Autodesk Fusion 360 part; units mm, degrees
note: some values were not read from the file. Set by a fixed rule: which face or edge a step refers to.
(part 2 of 4)
sketch "Sketch5" plane through (0, 0, -9.6) normal (0, 0, -1) x (1, 0, 0) in component "M5xxx-base"
  line L0 (101.4, -66.4) -> (-101.4, -66.4) construction
  line L1 (-101.4, -66.4) -> (-101.4, 66.4) construction
  line L2 (-101.4, 66.4) -> (101.4, 66.4) construction
  line L3 (101.4, 66.4) -> (101.4, -66.4) construction
  line L4 (101.4, -66.4) -> (-101.4, 66.4) construction
  line L5 (-101.4, -66.4) -> (101.4, 66.4) construction
  line L6 (113.4, -70) -> (113.4, 70) construction
  line L7 (-107, -78.4) -> (106, -78.4) construction
  circle A0 centre (101.4, -66.4) radius 6
  circle A1 centre (101.4, 66.4) radius 6
  circle A2 centre (0, 66.4) radius 6
  circle A3 centre (0, -66.4) radius 6
  circle A4 centre (-101.4, -66.4) radius 6
  circle A5 centre (-101.4, 66.4) radius 6
  line L8 (-82, 62) -> (-10, 62)
  line L9 (-10, 62) -> (-10, 15)
  line L10 (-15, 10) -> (-82, 10)
  line L11 (-87, 15) -> (-87, 57)
  line L12 (10, 15) -> (10, 57)
  line L13 (15, 62) -> (82, 62)
  line L14 (87, 57) -> (87, 15)
  line L15 (82, 10) -> (15, 10)
  line L16 (-87, -57) -> (-87, -15)
  line L17 (-82, -10) -> (-15, -10)
  line L18 (-10, -15) -> (-10, -57)
  line L19 (-15, -62) -> (-82, -62)
  line L20 (87, -62) -> (15, -62)
  line L21 (10, -57) -> (10, -15)
  line L22 (15, -10) -> (87, -10)
  line L23 (87, -10) -> (87, -62)
  arc A6 (-15, 10) -> (-10, 15) centre (-15, 15) ccw
  arc A7 (-87, 15) -> (-82, 10) centre (-82, 15) ccw
  arc A8 (-82, 62) -> (-87, 57) centre (-82, 57) ccw
  arc A9 (15, 62) -> (10, 57) centre (15, 57) ccw
  arc A10 (87, 57) -> (82, 62) centre (82, 57) ccw
  arc A11 (82, 10) -> (87, 15) centre (82, 15) ccw
  arc A12 (10, 15) -> (15, 10) centre (15, 15) ccw
  arc A13 (-82, -10) -> (-87, -15) centre (-82, -15) ccw
  arc A14 (-10, -15) -> (-15, -10) centre (-15, -15) ccw
  arc A15 (-15, -62) -> (-10, -57) centre (-15, -57) ccw
  arc A16 (-87, -57) -> (-82, -62) centre (-82, -57) ccw
  arc A17 (10, -57) -> (15, -62) centre (15, -57) ccw
  arc A18 (15, -10) -> (10, -15) centre (15, -15) ccw
  line L24 (-107, -76.4) -> (106, -76.4)
  line L25 (106, 76.4) -> (-107, 76.4)
  arc A19 (-107, 76.4) -> (-113.3999, 69.9694) centre (-107, 70) ccw
  line L26 (-113.3999, 69.9694) -> (-113.3999, -69.9694)
  arc A20 (-113.3999, -69.9694) -> (-107, -76.4) centre (-107, -70) ccw
  arc A21 (106, -76.4) -> (112.4, -70) centre (106, -70) ccw
  line L27 (112.4, -70) -> (112.4, 70)
  arc A22 (112.4, 70) -> (106, 76.4) centre (106, 70) ccw
  arc A23 (-113.3999, -69.9694) -> (-107, -76.4) centre (-107, -70) ccw
  line L28 (-107, -76.4) -> (106, -76.4)
  arc A24 (106, -76.4) -> (112.4, -70) centre (106, -70) ccw
  line L29 (112.4, -70) -> (112.4, 70)
  arc A25 (112.4, 70) -> (106, 76.4) centre (106, 70) ccw
  line L30 (106, 76.4) -> (-107, 76.4)
  arc A26 (-107, 76.4) -> (-113.3999, 69.9694) centre (-107, 70) ccw
  line L31 (-113.3999, 69.9694) -> (-113.3999, -69.9694)
  line L32 (80.7624, -50) -> (85.3812, -42)
  line L33 (85.3812, -42) -> (94.6188, -42)
  line L34 (94.6188, -42) -> (99.2376, -50)
  line L35 (99.2376, -50) -> (94.6188, -58)
  line L36 (94.6188, -58) -> (85.3812, -58)
  line L37 (85.3812, -58) -> (80.7624, -50)
  line L38 (80.7624, 50) -> (85.3812, 58)
  line L39 (85.3812, 58) -> (94.6188, 58)
  line L40 (94.6188, 58) -> (99.2376, 50)
  line L41 (99.2376, 50) -> (94.6188, 42)
  line L42 (94.6188, 42) -> (85.3812, 42)
  line L43 (85.3812, 42) -> (80.7624, 50)
  line L44 (50.7624, -25) -> (55.3812, -17)
  line L45 (55.3812, -17) -> (64.6188, -17)
  line L46 (64.6188, -17) -> (69.2376, -25)
  line L47 (69.2376, -25) -> (64.6188, -33)
  line L48 (64.6188, -33) -> (55.3812, -33)
  line L49 (55.3812, -33) -> (50.7624, -25)
  line L50 (20.7624, 0) -> (25.3812, 8)
  line L51 (25.3812, 8) -> (34.6188, 8)
  line L52 (34.6188, 8) -> (39.2376, 0)
  line L53 (39.2376, 0) -> (34.6188, -8)
  line L54 (34.6188, -8) -> (25.3812, -8)
  line L55 (25.3812, -8) -> (20.7624, 0)
  line L56 (-9.2376, 25) -> (-4.6188, 33)
  line L57 (-4.6188, 33) -> (4.6188, 33)
  line L58 (4.6188, 33) -> (9.2376, 25)
  line L59 (9.2376, 25) -> (4.6188, 17)
  line L60 (4.6188, 17) -> (-4.6188, 17)
  line L61 (-4.6188, 17) -> (-9.2376, 25)
  line L62 (-39.2376, -50) -> (-34.6188, -42)
  line L63 (-34.6188, -42) -> (-25.3812, -42)
  line L64 (-25.3812, -42) -> (-20.7624, -50)
  line L65 (-20.7624, -50) -> (-25.3812, -58)
  line L66 (-25.3812, -58) -> (-34.6188, -58)
  line L67 (-34.6188, -58) -> (-39.2376, -50)
  line L68 (-39.2376, 50) -> (-34.6188, 58)
  line L69 (-34.6188, 58) -> (-25.3812, 58)
  line L70 (-25.3812, 58) -> (-20.7624, 50)
  line L71 (-20.7624, 50) -> (-25.3812, 42)
  line L72 (-25.3812, 42) -> (-34.6188, 42)
  line L73 (-34.6188, 42) -> (-39.2376, 50)
  line L74 (-69.2376, -25) -> (-64.6188, -17)
  line L75 (-64.6188, -17) -> (-55.3812, -17)
  line L76 (-55.3812, -17) -> (-50.7624, -25)
  line L77 (-50.7624, -25) -> (-55.3812, -33)
  line L78 (-55.3812, -33) -> (-64.6188, -33)
  line L79 (-64.6188, -33) -> (-69.2376, -25)
  line L80 (-99.2376, 0) -> (-94.6188, 8)
  line L81 (-94.6188, 8) -> (-85.3812, 8)
  line L82 (-85.3812, 8) -> (-80.7624, 0)
  line L83 (-80.7624, 0) -> (-85.3812, -8)
  line L84 (-85.3812, -8) -> (-94.6188, -8)
  line L85 (-94.6188, -8) -> (-99.2376, 0)
  line L86 (-99.2376, 25) -> (-94.6188, 33)
  line L87 (-94.6188, 33) -> (-85.3812, 33)
  line L88 (-85.3812, 33) -> (-80.7624, 25)
  line L89 (-80.7624, 25) -> (-85.3812, 17)
  line L90 (-85.3812, 17) -> (-94.6188, 17)
  line L91 (-94.6188, 17) -> (-99.2376, 25)
  line L92 (-69.2376, -50) -> (-64.6188, -42)
  line L93 (-64.6188, -42) -> (-55.3812, -42)
  line L94 (-55.3812, -42) -> (-50.7624, -50)
  line L95 (-50.7624, -50) -> (-55.3812, -58)
  line L96 (-55.3812, -58) -> (-64.6188, -58)
  line L97 (-64.6188, -58) -> (-69.2376, -50)
  line L98 (-69.2376, 50) -> (-64.6188, 58)
  line L99 (-64.6188, 58) -> (-55.3812, 58)
  line L100 (-55.3812, 58) -> (-50.7624, 50)
  line L101 (-50.7624, 50) -> (-55.3812, 42)
  line L102 (-55.3812, 42) -> (-64.6188, 42)
  line L103 (-64.6188, 42) -> (-69.2376, 50)
  line L104 (-39.2376, -25) -> (-34.6188, -17)
  line L105 (-34.6188, -17) -> (-25.3812, -17)
  line L106 (-25.3812, -17) -> (-20.7624, -25)
  line L107 (-20.7624, -25) -> (-25.3812, -33)
  line L108 (-25.3812, -33) -> (-34.6188, -33)
  line L109 (-34.6188, -33) -> (-39.2376, -25)
  line L110 (4.6188, 8) -> (9.2376, 0)
  line L111 (9.2376, 0) -> (4.6188, -8)
  line L112 (4.6188, -8) -> (-4.6188, -8)
  line L113 (-4.6188, -8) -> (-9.2376, 0)
  line L114 (-9.2376, 0) -> (-4.6188, 8)
  line L115 (-4.6188, 8) -> (4.6188, 8)
  line L116 (20.7624, 25) -> (25.3812, 33)
  line L117 (25.3812, 33) -> (34.6188, 33)
  line L118 (34.6188, 33) -> (39.2376, 25)
  line L119 (39.2376, 25) -> (34.6188, 17)
  line L120 (34.6188, 17) -> (25.3812, 17)
  line L121 (25.3812, 17) -> (20.7624, 25)
  line L122 (50.7624, -50) -> (55.3812, -42)
  line L123 (55.3812, -42) -> (64.6188, -42)
  line L124 (64.6188, -42) -> (69.2376, -50)
  line L125 (69.2376, -50) -> (64.6188, -58)
  line L126 (64.6188, -58) -> (55.3812, -58)
  line L127 (55.3812, -58) -> (50.7624, -50)
  line L128 (50.7624, 50) -> (55.3812, 58)
  line L129 (55.3812, 58) -> (64.6188, 58)
  line L130 (64.6188, 58) -> (69.2376, 50)
  line L131 (69.2376, 50) -> (64.6188, 42)
  line L132 (64.6188, 42) -> (55.3812, 42)
  line L133 (55.3812, 42) -> (50.7624, 50)
  line L134 (80.7624, -25) -> (85.3812, -17)
  line L135 (85.3812, -17) -> (94.6188, -17)
  line L136 (94.6188, -17) -> (99.2376, -25)
  line L137 (99.2376, -25) -> (94.6188, -33)
  line L138 (94.6188, -33) -> (85.3812, -33)
  line L139 (85.3812, -33) -> (80.7624, -25)
  line L140 (80.7624, 25) -> (85.3812, 33)
  line L141 (85.3812, 33) -> (94.6188, 33)
  line L142 (94.6188, 33) -> (99.2376, 25)
  line L143 (99.2376, 25) -> (94.6188, 17)
  line L144 (94.6188, 17) -> (85.3812, 17)
  line L145 (85.3812, 17) -> (80.7624, 25)
  line L146 (50.7624, 0) -> (55.3812, 8)
  line L147 (55.3812, 8) -> (64.6188, 8)
  line L148 (64.6188, 8) -> (69.2376, 0)
  line L149 (69.2376, 0) -> (64.6188, -8)
  line L150 (64.6188, -8) -> (55.3812, -8)
  line L151 (55.3812, -8) -> (50.7624, 0)
  line L152 (20.7624, -25) -> (25.3812, -17)
  line L153 (25.3812, -17) -> (34.6188, -17)
  line L154 (34.6188, -17) -> (39.2376, -25)
  line L155 (39.2376, -25) -> (34.6188, -33)
  line L156 (34.6188, -33) -> (25.3812, -33)
  line L157 (25.3812, -33) -> (20.7624, -25)
  line L158 (-9.2376, 50) -> (-4.6188, 58)
  line L159 (-4.6188, 58) -> (4.6188, 58)
  line L160 (4.6188, 58) -> (9.2376, 50)
  line L161 (9.2376, 50) -> (4.6188, 42)
  line L162 (4.6188, 42) -> (-4.6188, 42)
  line L163 (-4.6188, 42) -> (-9.2376, 50)
  line L164 (-9.2376, -50) -> (-4.6188, -42)
  line L165 (-4.6188, -42) -> (4.6188, -42)
  line L166 (4.6188, -42) -> (9.2376, -50)
  line L167 (9.2376, -50) -> (4.6188, -58)
  line L168 (4.6188, -58) -> (-4.6188, -58)
  line L169 (-4.6188, -58) -> (-9.2376, -50)
  line L170 (-39.2376, 25) -> (-34.6188, 33)
  line L171 (-34.6188, 33) -> (-25.3812, 33)
  line L172 (-25.3812, 33) -> (-20.7624, 25)
  line L173 (-20.7624, 25) -> (-25.3812, 17)
  line L174 (-25.3812, 17) -> (-34.6188, 17)
  line L175 (-34.6188, 17) -> (-39.2376, 25)
  line L176 (-69.2376, 0) -> (-64.6188, 8)
  line L177 (-64.6188, 8) -> (-55.3812, 8)
  line L178 (-55.3812, 8) -> (-50.7624, 0)
  line L179 (-50.7624, 0) -> (-55.3812, -8)
  line L180 (-55.3812, -8) -> (-64.6188, -8)
  line L181 (-64.6188, -8) -> (-69.2376, 0)
  line L182 (-99.2376, -25) -> (-94.6188, -17)
  line L183 (-94.6188, -17) -> (-85.3812, -17)
  line L184 (-85.3812, -17) -> (-80.7624, -25)
  line L185 (-80.7624, -25) -> (-85.3812, -33)
  line L186 (-85.3812, -33) -> (-94.6188, -33)
  line L187 (-94.6188, -33) -> (-99.2376, -25)
  line L188 (-99.2376, 50) -> (-94.6188, 58)
  line L189 (-94.6188, 58) -> (-85.3812, 58)
  line L190 (-85.3812, 58) -> (-80.7624, 50)
  line L191 (-80.7624, 50) -> (-85.3812, 42)
  line L192 (-85.3812, 42) -> (-94.6188, 42)
  line L193 (-94.6188, 42) -> (-99.2376, 50)
  line L194 (-99.2376, -50) -> (-94.6188, -42)
  line L195 (-94.6188, -42) -> (-85.3812, -42)
  line L196 (-85.3812, -42) -> (-80.7624, -50)
  line L197 (-80.7624, -50) -> (-85.3812, -58)
  line L198 (-85.3812, -58) -> (-94.6188, -58)
  line L199 (-94.6188, -58) -> (-99.2376, -50)
  line L200 (-69.2376, 25) -> (-64.6188, 33)
  line L201 (-64.6188, 33) -> (-55.3812, 33)
  line L202 (-55.3812, 33) -> (-50.7624, 25)
  line L203 (-50.7624, 25) -> (-55.3812, 17)
  line L204 (-55.3812, 17) -> (-64.6188, 17)
  line L205 (-64.6188, 17) -> (-69.2376, 25)
  line L206 (-39.2376, 0) -> (-34.6188, 8)
  line L207 (-34.6188, 8) -> (-25.3812, 8)
  line L208 (-25.3812, 8) -> (-20.7624, 0)
  line L209 (-20.7624, 0) -> (-25.3812, -8)
  line L210 (-25.3812, -8) -> (-34.6188, -8)
  line L211 (-34.6188, -8) -> (-39.2376, 0)
  line L212 (-9.2376, -25) -> (-4.6188, -17)
  line L213 (-4.6188, -17) -> (4.6188, -17)
  line L214 (4.6188, -17) -> (9.2376, -25)
  line L215 (9.2376, -25) -> (4.6188, -33)
  line L216 (4.6188, -33) -> (-4.6188, -33)
  line L217 (-4.6188, -33) -> (-9.2376, -25)
  line L218 (20.7624, 50) -> (25.3812, 58)
  line L219 (25.3812, 58) -> (34.6188, 58)
  line L220 (34.6188, 58) -> (39.2376, 50)
  line L221 (39.2376, 50) -> (34.6188, 42)
  line L222 (34.6188, 42) -> (25.3812, 42)
  line L223 (25.3812, 42) -> (20.7624, 50)
  line L224 (20.7624, -50) -> (25.3812, -42)
  line L225 (25.3812, -42) -> (34.6188, -42)
  line L226 (34.6188, -42) -> (39.2376, -50)
  line L227 (39.2376, -50) -> (34.6188, -58)
  line L228 (34.6188, -58) -> (25.3812, -58)
  line L229 (25.3812, -58) -> (20.7624, -50)
  line L230 (50.7624, 25) -> (55.3812, 33)
  line L231 (55.3812, 33) -> (64.6188, 33)
  line L232 (64.6188, 33) -> (69.2376, 25)
  line L233 (69.2376, 25) -> (64.6188, 17)
  line L234 (64.6188, 17) -> (55.3812, 17)
  line L235 (55.3812, 17) -> (50.7624, 25)
  line L236 (80.7624, 0) -> (85.3812, 8)
  line L237 (85.3812, 8) -> (94.6188, 8)
  line L238 (94.6188, 8) -> (99.2376, 0)
  line L239 (99.2376, 0) -> (94.6188, -8)
  line L240 (94.6188, -8) -> (85.3812, -8)
  line L241 (85.3812, -8) -> (80.7624, 0)
  dimension "d116" = 12
  dimension "d117" = 12
  dimension "d118" = 12
  constraint perpendicular L0 L1
  constraint parallel L0 L2
  constraint parallel L1 L3
  constraint horizontal L0
  constraint coincident L4 origin
  constraint coincident L5 origin
  constraint coincident L0.start L3.end
  constraint coincident L2.end L3.start
  constraint midpoint L2 A2.centre
  constraint midpoint L0 A3.centre
  constraint coincident L0.end L1.start
  constraint coincident L1.end L2.start
  constraint equal A3 A4
  constraint equal A0 A3
  constraint equal A0 A1
  constraint equal A1 A2
  constraint equal A2 A5
  measures "d116" distance of L3 L6
  measures "d117" distance of L0 L7
  measures "d118" diameter of A0
extrude "Extrude9" cut sketch "Sketch5" against normal blind 0.6 contours A0 | A1 | A2 | A3 | A4 | A5 bodies 3 in component "M5xxx-base"
combine "Combine1" operation cut target body 3 tool bodies 2 1 1 body 1 seen with x (1, 0, 0) y (0, 1, 0) z (0, 0, 1) at (0, 0, 16.6) body 1 seen with x (1, 0, 0) y (0, 1, 0) z (0, 0, 1) at (0, 0, 0) keep tools in component "M5xxx-base"
move_face "OffsetFaces1" offset -2 2 faces at (112.1333, -45.5056, 23.3243) (112.1333, -45.5056, 6.7243) on bodies 3 in component "M5xxx-base"
sketch "Sketch11" plane through (0, 0, 34.2) normal (0, 0, 1) x (-1, 0, 0) in component "M5xxx-base"
  line L0 (-88.8, 76) -> (-41.2, 76)
  line L1 (-41.2, 76) -> (-41.2, 78.4)
  line L2 (-41.2, 78.4) -> (-88.8, 78.4)
  line L3 (-88.8, 78.4) -> (-88.8, 76)
  line L4 (-65.4, 78.4) -> (-64.6, 78.4)
  line L5 (-64.6, 78.4) -> (-64.6, 76)
  line L6 (-64.6, 76) -> (-65.4, 76)
  line L7 (-65.4, 76) -> (-65.4, 78.4)
  line L8 (-65.4, 78.4) -> (-64.6, 76) construction
  line L9 (-64.6, 78.4) -> (-65.4, 76) construction
  line L10 (-65, 77.2) -> (-65, 76) construction
  point P0 (-65, 77.2)
  dimension "d193" = 0.8
  constraint perpendicular L4 L5
  constraint parallel L4 L6
  constraint parallel L5 L7
  constraint horizontal L4
  constraint coincident L2 L4.start
  constraint coincident L8 P0
  constraint coincident L9 P0
  constraint coincident L0 L6.end
  constraint coincident P0 L10.start
  constraint midpoint L0 L10.end
  constraint vertical L10
  measures "d193" distance of L5.end L6.end
extrude "Extrude17" add sketch "Sketch11" along normal blind 19 contours L0 L2 L4 L5 L6 L7 bodies 3 in component "M5xxx-base"
sketch "Sketch8" plane through (0, 0, -1.6) normal (0, 0, 1) x (-1, 0, 0) in component "M5xxx-base"
  line L0 (-111, 16.2) -> (-114.4, 16.2)
  line L1 (-114.4, 16.2) -> (-114.4, 15.4)
  line L2 (-114.4, 15.4) -> (-111, 15.4)
  line L3 (-111, 15.4) -> (-111, 16.2)
  line L4 (-111, 0.4) -> (-114.4, 0.4)
  line L5 (-114.4, 0.4) -> (-114.4, -0.4)
  line L6 (-114.4, -0.4) -> (-111, -0.4)
  line L7 (-111, -0.4) -> (-111, 0.4)
  line L8 (-111, -15.4) -> (-114.4, -15.4)
  line L9 (-114.4, -15.4) -> (-114.4, -16.2)
  line L10 (-114.4, -16.2) -> (-111, -16.2)
  line L11 (-111, -16.2) -> (-111, -15.4)
  line L12 (-111, 0) -> (-114.4, 0) construction
  circle A0 centre (-105, -70) radius 5
  line L13 (-106.5, -70) -> (-105.75, -68.701)
  line L14 (-105.75, -68.701) -> (-104.25, -68.701)
  line L15 (-104.25, -68.701) -> (-103.5, -70)
  line L16 (-103.5, -70) -> (-104.25, -71.299)
  line L17 (-104.25, -71.299) -> (-105.75, -71.299)
  line L18 (-105.75, -71.299) -> (-106.5, -70)
  circle A1 centre (-15, 70) radius 5
  line L19 (-15.75, 68.701) -> (-16.5, 70)
  line L20 (-16.5, 70) -> (-15.75, 71.299)
  line L21 (-15.75, 71.299) -> (-14.25, 71.299)
  line L22 (-14.25, 71.299) -> (-13.5, 70)
  line L23 (-13.5, 70) -> (-14.25, 68.701)
  line L24 (-14.25, 68.701) -> (-15.75, 68.701)
  circle A2 centre (105, -70) radius 5
  line L25 (104.25, -71.299) -> (103.5, -70)
  line L26 (103.5, -70) -> (104.25, -68.701)
  line L27 (104.25, -68.701) -> (105.75, -68.701)
  line L28 (105.75, -68.701) -> (106.5, -70)
  line L29 (106.5, -70) -> (105.75, -71.299)
  line L30 (105.75, -71.299) -> (104.25, -71.299)
  circle A3 centre (105, 70) radius 5
  line L31 (104.25, 68.701) -> (103.5, 70)
  line L32 (103.5, 70) -> (104.25, 71.299)
  line L33 (104.25, 71.299) -> (105.75, 71.299)
  line L34 (105.75, 71.299) -> (106.5, 70)
  line L35 (106.5, 70) -> (105.75, 68.701)
  line L36 (105.75, 68.701) -> (104.25, 68.701)
  circle A4 centre (-105, 70) radius 5
  line L37 (-105.75, 71.299) -> (-104.25, 71.299)
  line L38 (-104.25, 71.299) -> (-103.5, 70)
  line L39 (-103.5, 70) -> (-104.25, 68.701)
  line L40 (-104.25, 68.701) -> (-105.75, 68.701)
  line L41 (-105.75, 68.701) -> (-106.5, 70)
  line L42 (-106.5, 70) -> (-105.75, 71.299)
  dimension "d134" = 0.8
  dimension "d135" = 15
  constraint horizontal L0
  constraint vertical L1
  constraint horizontal L2
  constraint vertical L3
  constraint horizontal L4
  constraint vertical L5
  constraint horizontal L6
  constraint vertical L7
  constraint horizontal L8
  constraint vertical L9
  constraint horizontal L10
  constraint vertical L11
  constraint equal L7 L11
  constraint equal L3 L7
  constraint midpoint L7 L12.start
  constraint midpoint L5 L12.end
  constraint horizontal origin L12.start
  constraint symmetric L1.end L8.end L12
  measures "d134" distance of L0.start L2.end
  measures "d135" distance of L5.end L8.end
extrude "Extrude12" add sketch "Sketch8" along normal blind 44.8 contours L0 L1 L2 L3 | L4 L5 L6 L7 | L8 L9 L10 L11 bodies 3 in component "M5xxx-base"
chamfer "Chamfer7" distance 0.4 angle 45 41 edges at (114.4, -15.4, 37.4) (114.4, 0.4, 37.4) (114.4, 0.4, 37.4) (114.4, 0.4, 5.2) (114.4, 0.4, 21.8) (114.4, -15.4, 21.8) (114.4, -15.4, 5.2) (114.4, -15.4, 37.4) (114.4, 0.4, 37.4) (114.4, 0.4, 5.2) (114.4, 0.4, 21.8) (114.4, -15.4, 21.8) (114.4, -15.4, 5.2) (114.4, -15.4, 37.4) (114.4, 16.2, 37.4) (114.4, 16.2, 5.2) (114.4, 16.2, 21.8) (114.4, 16.2, 37.4) (114.4, 16.2, 5.2) (114.4, 16.2, 21.8) (114.4, 16.2, 37.4) (111, 15.4, 5.2) (111, 15.4, 37.4) (111, 15.4, 21.8) (111, 15.4, 5.2) (111, 15.4, 37.4) (111, 15.4, 21.8) (111, -0.4, 21.8) (111, -0.4, 37.4) (111, -0.4, 5.2) (111, -16.2, 5.2) (111, -16.2, 21.8) (111, -16.2, 37.4) (111, -16.2, 5.2) (111, -16.2, 21.8) (111, -16.2, 37.4) (111, -16.2, 37.4) (111, -0.4, 37.4) (111, 15.4, 37.4) (65.4, -78.4, 43.7) (64.6, -76, 43.7) measured on face at (114.4, 52, 12.8214) measured on face at (114.4, 52, 12.8214) measured on face at (114.4, 52, 12.8214) measured on face at (114.4, 52, 12.8214) measured on face at (114.4, 52, 12.8214) measured on face at (114.4, 52, 12.8214) measured on face at (114.4, 52, 12.8214) measured on face at (114.4, 52, 12.8214) measured on face at (114.4, 52, 12.8214) measured on face at (114.4, 52, 12.8214) measured on face at (114.4, 52, 12.8214) measured on face at (114.4, 52, 12.8214) measured on face at (114.4, 52, 12.8214) measured on face at (114.4, 52, 12.8214) measured on face at (114.4, 52, 12.8214) measured on face at (114.4, 52, 12.8214) measured on face at (114.4, 52, 12.8214) measured on face at (114.4, 52, 12.8214) measured on face at (114.4, 52, 12.8214) measured on face at (114.4, 52, 12.8214) measured on face at (114.4, 52, 12.8214) measured on face at (111, 52, 13.6667) measured on face at (111, 52, 13.6667) measured on face at (111, 52, 13.6667) measured on face at (111, 52, 13.6667) measured on face at (111, 52, 13.6667) measured on face at (111, 52, 13.6667) measured on face at (111, 52, 13.6667) measured on face at (111, 52, 13.6667) measured on face at (111, 52, 13.6667) measured on face at (111, 52, 13.6667) measured on face at (111, 52, 13.6667) measured on face at (111, 52, 13.6667) measured on face at (111, 52, 13.6667) measured on face at (111, 52, 13.6667) measured on face at (111, 52, 13.6667) measured on face at (111, 52, 13.6667) measured on face at (111, 52, 13.6667) measured on face at (111, 52, 13.6667) measured on face at (-64.8175, -78.4, 31.9138) measured on face at (-64.8175, -76, 32.7591) on bodies 3 in component "M5xxx-base"
sketch "Sketch7" plane through (114.4, 0, 0) normal (1, 0, 0) x (0, 1, 0) in component "M5xxx-base"
  line L0 (70, -6.1359) -> (70, 58.4)
  line L1 (70, 58.4) -> (-70, 58.4)
  line L2 (-70, 58.4) -> (-70, -6.1359)
  circle A0 centre (50, 7.5) radius 6.4
  line L3 (-61.6, 16.6) -> (-70, 16.6)
  line L4 (-75, 16.6) -> (-70, 16.6)
  line L5 (-75, 16.6) -> (-70, 16.6)
  line L6 (-70, 16.6) -> (-56, 16.6)
  line L7 (-56, 16.6) -> (-44, 16.6)
  line L8 (-44, 16.6) -> (-32, 16.6)
  line L9 (-58.4, 16.6) -> (-61.6, 16.6)
  line L10 (-71.75, 16.6) -> (-68.25, 16.6)
  line L11 (-71.75, 16.6) -> (-68.25, 16.6)
  line L12 (-71.75, 16.6) -> (-68.25, 16.6)
  line L13 (78.4, 58.4) -> (78.4, -6.1359)
  line L14 (50, 7.5) -> (56.4, 7.5) construction
  line L15 (47.7729, 13.5) -> (52.2271, 13.5)
  line L16 (47.7729, 1.5) -> (52.2271, 1.5)
  circle A1 centre (50, 7.5) radius 8
  line L17 (57.7859, 5.6614) -> (55, -6.1359)
  line L18 (42.2141, 5.6614) -> (45, -6.1359)
  line L19 (50, 7.5) -> (50, -6.1359) construction
  line L20 (46, 33.2) -> (54, 33.2)
  line L21 (50, 7.5) -> (50, 33.2) construction
  line L22 (15.8, 44) -> (32, 44)
  line L23 (32, 44) -> (32, 32.4)
  line L24 (32, 32.4) -> (15.8, 32.4)
  line L25 (15.8, 32.4) -> (15.8, 44)
  line L26 (15.8, 27) -> (32, 27)
  line L27 (32, 27) -> (32, 15.8)
  line L28 (32, 15.8) -> (15.8, 15.8)
  line L29 (15.8, 15.8) -> (15.8, 27)
  line L30 (15.8, 10.4) -> (32, 10.4)
  line L31 (32, 10.4) -> (32, -0.8)
  line L32 (32, -0.8) -> (15.8, -0.8)
  line L33 (15.8, -0.8) -> (15.8, 10.4)
  line L34 (-15.8, 10.4) -> (-0.4, 10.4)
  line L35 (-0.4, 10.4) -> (-0.4, -0.8)
  line L36 (-15.8, -0.8) -> (-15.8, 10.4)
  line L37 (0, 10.4) -> (15.4, 10.4)
  line L38 (15.4, 10.4) -> (15.4, -0.8)
  line L39 (0, -0.8) -> (0, 10.4)
  line L40 (-15.8, 27) -> (-0.4, 27)
  line L41 (-0.4, 27) -> (-0.4, 15.8)
  line L42 (-15.8, 15.8) -> (-15.8, 27)
  line L43 (0, 27) -> (15.4, 27)
  line L44 (15.4, 27) -> (15.4, 15.8)
  line L45 (0, 15.8) -> (0, 27)
  line L46 (0, 44) -> (15.4, 44)
  line L47 (15.4, 44) -> (15.4, 32.4)
  line L48 (0, 32.4) -> (0, 44)
  line L49 (-15.8, 44) -> (-0.4, 44)
  line L50 (-0.4, 44) -> (-0.4, 32.4)
  line L51 (-15.8, 32.4) -> (-15.8, 44)
  line L52 (-32, -0.8) -> (-32, 10.4)
  line L53 (-32, 10.4) -> (-16.2, 10.4)
  line L54 (-16.2, 10.4) -> (-16.2, -0.8)
  line L55 (-32, 15.8) -> (-32, 27)
  line L56 (-32, 27) -> (-16.2, 27)
  line L57 (-16.2, 27) -> (-16.2, 15.8)
  line L58 (-16.2, 44) -> (-16.2, 32.4)
  line L59 (-32, 32.4) -> (-32, 44)
  line L60 (-32, 44) -> (-16.2, 44)
  line L61 (-70, -6.1359) -> (70, -6.1359)
  line L62 (70, -6.1359) -> (70, 58.4)
  line L63 (70, 58.4) -> (-70, 58.4)
  line L64 (-70, 58.4) -> (-70, -6.1359)
  arc A2 (54, 34.2) -> (59, 39.2) centre (54, 39.2) ccw
  line L65 (54, 34.2) -> (46, 34.2)
  arc A3 (41, 39.2) -> (46, 34.2) centre (46, 39.2) ccw
  line L66 (41, 39.2) -> (41, 48.2)
  arc A4 (46, 53.2) -> (41, 48.2) centre (46, 48.2) ccw
  line L67 (46, 53.2) -> (54, 53.2)
  arc A5 (59, 48.2) -> (54, 53.2) centre (54, 48.2) ccw
  line L68 (59, 48.2) -> (59, 39.2)
  circle A6 centre (-50, 24.1) radius 6.5
  circle A7 centre (-50, 7.5) radius 6.5
  line L69 (45, -6.1359) -> (55, -6.1359)
  line L70 (-0.4, -0.8) -> (-15.8, -0.8)
  line L71 (15.4, -0.8) -> (0, -0.8)
  line L72 (-0.4, 15.8) -> (-15.8, 15.8)
  line L73 (15.4, 15.8) -> (0, 15.8)
  line L74 (-16.2, -0.8) -> (-32, -0.8)
  line L75 (-16.2, 15.8) -> (-32, 15.8)
  line L76 (15.4, 32.4) -> (0, 32.4)
  line L77 (-0.4, 32.4) -> (-15.8, 32.4)
  line L78 (-16.2, 32.4) -> (-32, 32.4)
  line L79 (15.4, 32.4) -> (15.8, 32.4)
  line L80 (15.8, 32.4) -> (15.8, 44)
  line L81 (15.4, 15.8) -> (15.8, 15.8)
  line L82 (15.8, 15.8) -> (15.8, 27)
  line L83 (15.4, -0.8) -> (15.8, -0.8)
  line L84 (15.8, -0.8) -> (15.8, 10.4)
  line L85 (0, 10.4) -> (-0.4, 10.4)
  line L86 (-0.4, 10.4) -> (-0.4, -0.8)
  line L87 (-16.2, -0.8) -> (-15.8, -0.8)
  line L88 (-15.8, -0.8) -> (-15.8, 10.4)
  line L89 (15.8, 10.4) -> (15.4, 10.4)
  line L90 (15.4, 10.4) -> (15.4, -0.8)
  line L91 (-0.4, -0.8) -> (0, -0.8)
  line L92 (0, -0.8) -> (0, 10.4)
  line L93 (0, 27) -> (-0.4, 27)
  line L94 (-0.4, 27) -> (-0.4, 15.8)
  line L95 (-16.2, 15.8) -> (-15.8, 15.8)
  line L96 (-15.8, 15.8) -> (-15.8, 27)
  line L97 (15.8, 27) -> (15.4, 27)
  line L98 (15.4, 27) -> (15.4, 15.8)
  line L99 (-0.4, 15.8) -> (0, 15.8)
  line L100 (0, 15.8) -> (0, 27)
  line L101 (15.8, 44) -> (15.4, 44)
  line L102 (15.4, 44) -> (15.4, 32.4)
  line L103 (-0.4, 32.4) -> (0, 32.4)
  line L104 (0, 32.4) -> (0, 44)
  line L105 (0, 44) -> (-0.4, 44)
  line L106 (-0.4, 44) -> (-0.4, 32.4)
  line L107 (-16.2, 32.4) -> (-15.8, 32.4)
  line L108 (-15.8, 32.4) -> (-15.8, 44)
  line L109 (-15.8, 10.4) -> (-16.2, 10.4)
  line L110 (-16.2, 10.4) -> (-16.2, -0.8)
  line L111 (-15.8, 27) -> (-16.2, 27)
  line L112 (-16.2, 27) -> (-16.2, 15.8)
  line L113 (-16.2, 44) -> (-16.2, 32.4)
  line L114 (-15.8, 44) -> (-16.2, 44)
  line L115 (75, 0) -> (-75, 0)
  circle A8 centre (-50, 6.5) radius 6.5
  line L116 (-32, 0) -> (-32, 10.4)
  line L117 (15.8, 10.4) -> (32, 10.4)
  line L118 (32, 10.4) -> (32, 0)
  circle A9 centre (-50, 23.1) radius 6.5
  line L119 (-32, 16.6) -> (-32, 27)
  line L120 (15.8, 27) -> (32, 27)
  line L121 (32, 27) -> (32, 16.6)
  arc A10 (54, 34.2) -> (59, 39.2) centre (54, 39.2) ccw
  line L122 (54, 34.2) -> (46, 34.2)
  arc A11 (41, 39.2) -> (46, 34.2) centre (46, 39.2) ccw
  line L123 (41, 39.2) -> (41, 48.2)
  arc A12 (46, 53.2) -> (41, 48.2) centre (46, 48.2) ccw
  line L124 (46, 53.2) -> (54, 53.2)
  arc A13 (59, 48.2) -> (54, 53.2) centre (54, 48.2) ccw
  line L125 (59, 48.2) -> (59, 39.2)
  line L126 (32, 43.6) -> (32, 31.6)
  line L127 (32, 31.6) -> (15.8, 31.6)
  line L128 (-32, 31.6) -> (-32, 43.6)
  line L129 (-32, 43.6) -> (32, 43.6)
  line L130 (-70, -6.1359) -> (70, -6.1359)
  line L131 (70, -6.1359) -> (70, 58.4)
  line L132 (70, 58.4) -> (-70, 58.4)
  line L133 (-70, 58.4) -> (-70, -6.1359)
  line L134 (15.8, 31.6) -> (15.8, 43.2)
  line L135 (15.8, 16.6) -> (15.8, 27)
  line L136 (15.8, 0) -> (15.8, 10.4)
  line L137 (-15.8, 10.4) -> (-0.4, 10.4)
  line L138 (-0.4, 10.4) -> (-0.4, 0)
  line L139 (-15.8, 31.6) -> (-15.8, 43.2)
  line L140 (0, 10.4) -> (15.4, 10.4)
  line L141 (15.4, 10.4) -> (15.4, 0)
  line L142 (0, 31.6) -> (0, 43.2)
  line L143 (-15.8, 27) -> (-0.4, 27)
  line L144 (-15.8, 16.6) -> (-15.8, 27)
  line L145 (0, 27) -> (15.4, 27)
  line L146 (0, 16.6) -> (0, 27)
  line L147 (15.4, 43.2) -> (15.4, 31.6)
  line L148 (15.4, 31.6) -> (0, 31.6)
  line L149 (-0.4, 43.2) -> (-0.4, 31.6)
  line L150 (-0.4, 31.6) -> (-15.8, 31.6)
  line L151 (-32, 10.4) -> (-16.2, 10.4)
  line L152 (-16.2, 10.4) -> (-16.2, 0)
  line L153 (-32, 27) -> (-16.2, 27)
  line L154 (-16.2, 43.2) -> (-16.2, 31.6)
  line L155 (-16.2, 31.6) -> (-32, 31.6)
  line L156 (15.8, 43.2) -> (15.4, 43.2)
  line L157 (0, 43.2) -> (-0.4, 43.2)
  line L158 (-15.8, 43.2) -> (-16.2, 43.2)
  line L159 (32, 16.6) -> (15.8, 16.6)
  line L160 (32, 0) -> (15.8, 0)
  line L161 (-0.4, 0) -> (-15.8, 0)
  line L162 (-15.8, 0) -> (-15.8, 10.4)
  line L163 (-0.4, 27) -> (-0.4, 16.6)
  line L164 (-0.4, 16.6) -> (-15.8, 16.6)
  line L165 (15.4, 0) -> (0, 0)
  line L166 (0, 0) -> (0, 10.4)
  line L167 (15.4, 27) -> (15.4, 16.6)
  line L168 (15.4, 16.6) -> (0, 16.6)
  line L169 (-16.2, 0) -> (-32, 0)
  line L170 (-16.2, 16.6) -> (-32, 16.6)
  line L171 (-16.2, 27) -> (-16.2, 16.6)
  dimension "d123" = 12
  dimension "d124" = 12.8
  dimension "d127" = 16
  dimension "d128" = 10
  dimension "d200" = 7.5
  constraint coincident A0.centre L14.start
  constraint coincident A0 L14.end
  constraint horizontal L14
  constraint coincident A0 L15.start
  constraint coincident A0 L15.end
  constraint horizontal L15
  constraint coincident A0 L16.start
  constraint coincident A0 L16.end
  constraint parallel L15 L16
  constraint symmetric L14 L15.end L16.end
  constraint concentric A0 A1
  constraint coincident A1 L17.start
  constraint coincident A1 L18.start
  constraint tangent A1 L18
  constraint tangent A1 L17
  constraint symmetric L17.end L18.end L19
  constraint midpoint L20 L21.end
  constraint perpendicular L20 L21
  constraint vertical L19
  constraint midpoint L19.end L69
  constraint coincident L17.end L61
  measures "d123" distance of L15 L16
  measures "d124" diameter of A0
  measures "d127" diameter of A1
  measures "d128" distance of L17.end L18.end
  measures "d200" distance of A0.centre L115
extrude "Extrude14" add sketch "Sketch7" along normal blind 2.4 contours A1 L17 L18 L61 L69 L115 L130 | A1 L17 L115 | A1 L115 | A1 L115 | A1 L18 L115 | A0 L15 | A0 L16 bodies 3 in component "M5xxx-base"
extrude "Extrude15" cut sketch "Sketch7" against normal blind 11 contours A0 L15 L16 bodies 3 in component "M5xxx-base"
sketch "Sketch12" plane through (111, 0, 0) normal (-1, 0, 0) x (0, -1, 0) in component "M5xxx-base"
  line L0 (-47.7729, 1.5) -> (-52.2271, 1.5)
  arc A0 (-52.2271, 13.5) -> (-52.2271, 1.5) centre (-50, 7.5) ccw
  line L1 (-52.2271, 13.5) -> (-47.7729, 13.5)
  arc A1 (-47.7729, 1.5) -> (-47.7729, 13.5) centre (-50, 7.5) ccw
  line L2 (-0.4, 43.2) -> (-0.4, 31.6)
  line L3 (-0.4, 31.6) -> (-15.8, 31.6)
  line L4 (-15.8, 31.6) -> (-15.8, 43.2)
  line L5 (15.4, 43.2) -> (15.4, 31.6)
  line L6 (15.4, 31.6) -> (0, 31.6)
  line L7 (0, 31.6) -> (0, 43.2)
  line L8 (32, 43.6) -> (32, 31.6)
  line L9 (32, 31.6) -> (15.8, 31.6)
  line L10 (15.8, 31.6) -> (15.8, 43.2)
  line L11 (15.8, 10.4) -> (32, 10.4)
  line L12 (32, 10.4) -> (32, 0)
  line L13 (15.8, 0) -> (15.8, 10.4)
  line L14 (15.8, 27) -> (32, 27)
  line L15 (32, 27) -> (32, 16.6)
  line L16 (15.8, 16.6) -> (15.8, 27)
  line L17 (0, 27) -> (15.4, 27)
  line L18 (0, 16.6) -> (0, 27)
  line L19 (-15.8, 27) -> (-0.4, 27)
  line L20 (-15.8, 16.6) -> (-15.8, 27)
  line L21 (-15.8, 10.4) -> (-0.4, 10.4)
  line L22 (-15.8, 0) -> (-15.8, 10.4)
  line L23 (-32, 0) -> (-32, 10.4)
  line L24 (-32, 10.4) -> (-16.2, 10.4)
  line L25 (-16.2, 27) -> (-16.2, 16.6)
  line L26 (-32, 16.6) -> (-32, 27)
  line L27 (-32, 27) -> (-16.2, 27)
  line L28 (-16.2, 43.2) -> (-16.2, 31.6)
  line L29 (-16.2, 31.6) -> (-32, 31.6)
  line L30 (-32, 31.6) -> (-32, 43.6)
  line L31 (-32, 43.6) -> (32, 43.6)
  circle A2 centre (50, 6.5) radius 6.5
  circle A3 centre (50, 23.1) radius 6.5
  arc A4 (-59, 39.2) -> (-54, 34.2) centre (-54, 39.2) ccw
  line L32 (-59, 39.2) -> (-59, 48.2)
  arc A5 (-54, 53.2) -> (-59, 48.2) centre (-54, 48.2) ccw
  line L33 (-54, 53.2) -> (-46, 53.2)
  arc A6 (-41, 48.2) -> (-46, 53.2) centre (-46, 48.2) ccw
  line L34 (-41, 48.2) -> (-41, 39.2)
  arc A7 (-46, 34.2) -> (-41, 39.2) centre (-46, 39.2) ccw
  line L35 (-46, 34.2) -> (-54, 34.2)
  line L36 (-70, -3.6) -> (70, -3.6)
  line L37 (70, -3.6) -> (70, 58.4)
  line L38 (70, 58.4) -> (-70, 58.4)
  line L39 (-70, 58.4) -> (-70, -3.6)
  circle A8 centre (-50, 7.5) radius 8.5
  line L40 (32, 0) -> (15.8, 0)
  line L41 (15.8, 43.2) -> (15.4, 43.2)
  line L42 (0, 43.2) -> (-0.4, 43.2)
  line L43 (-15.8, 43.2) -> (-16.2, 43.2)
  line L44 (32, 16.6) -> (15.8, 16.6)
  line L45 (0, 10.4) -> (15.4, 10.4)
  line L46 (15.4, 10.4) -> (15.4, 0)
  line L47 (15.4, 0) -> (0, 0)
  line L48 (0, 0) -> (0, 10.4)
  line L49 (15.4, 27) -> (15.4, 16.6)
  line L50 (15.4, 16.6) -> (0, 16.6)
  line L51 (-16.2, 16.6) -> (-32, 16.6)
  line L52 (-16.2, 0) -> (-32, 0)
  line L53 (-16.2, 10.4) -> (-16.2, 0)
  line L54 (-0.4, 10.4) -> (-0.4, 0)
  line L55 (-0.4, 0) -> (-15.8, 0)
  line L56 (-0.4, 27) -> (-0.4, 16.6)
  line L57 (-0.4, 16.6) -> (-15.8, 16.6)
  dimension "d201" = 17
  constraint concentric A0 A8
  measures "d201" diameter of A8
extrude "Extrude18" cut sketch "Sketch12" against normal blind 2.4 contours A8 bodies 3 in component "M5xxx-base"
chamfer "Chamfer14" distance 4 angle 30 1 edges at (116.8, 50, -6.1359) measured on face at (116.8, 50.7424, -3.5906) on bodies 3 in component "M5xxx-base"
sketch "Sketch14" plane through (-115.3999, 0, 0) normal (-1, 0, 0) x (0, -1, 0) in component "M5xxx-base"
  circle A0 centre (60, 7.5) radius 1.75
  circle A1 centre (60, 24.1) radius 1.75
  line L0 (-69.9653, -6.1359) -> (69.9653, -6.1359)
  line L1 (69.9653, -6.1359) -> (69.9653, 58.4)
  line L2 (69.9653, 58.4) -> (-69.9653, 58.4)
  line L3 (-69.9653, 58.4) -> (-69.9653, -6.1359)
  line L4 (0, 0) -> (0, 58.4) construction
  line L5 (6.9282, 22.6) -> (3.4641, 28.6)
  line L6 (3.4641, 28.6) -> (-3.4641, 28.6)
  line L7 (-3.4641, 28.6) -> (-6.9282, 22.6)
  line L8 (-6.9282, 22.6) -> (-3.4641, 16.6)
  line L9 (-3.4641, 16.6) -> (3.4641, 16.6)
  line L10 (3.4641, 16.6) -> (6.9282, 22.6)
  line L11 (-26.5359, 12) -> (-33.4641, 12)
  line L12 (-33.4641, 12) -> (-36.9282, 6)
  line L13 (-36.9282, 6) -> (-33.4641, 0)
  line L14 (-33.4641, 0) -> (-26.5359, 0)
  line L15 (-26.5359, 0) -> (-23.0718, 6)
  line L16 (-23.0718, 6) -> (-26.5359, 12)
  line L17 (3.4641, 12) -> (-3.4641, 12)
  line L18 (-3.4641, 12) -> (-6.9282, 6)
  line L19 (-6.9282, 6) -> (-3.4641, 0)
  line L20 (-3.4641, 0) -> (3.4641, 0)
  line L21 (3.4641, 0) -> (6.9282, 6)
  line L22 (6.9282, 6) -> (3.4641, 12)
  line L23 (33.4641, 12) -> (26.5359, 12)
  line L24 (26.5359, 12) -> (23.0718, 6)
  line L25 (23.0718, 6) -> (26.5359, 0)
  line L26 (26.5359, 0) -> (33.4641, 0)
  line L27 (33.4641, 0) -> (36.9282, 6)
  line L28 (36.9282, 6) -> (33.4641, 12)
  line L29 (-26.5359, 28.6) -> (-33.4641, 28.6)
  line L30 (-33.4641, 28.6) -> (-36.9282, 22.6)
  line L31 (-36.9282, 22.6) -> (-33.4641, 16.6)
  line L32 (-33.4641, 16.6) -> (-26.5359, 16.6)
  line L33 (-26.5359, 16.6) -> (-23.0718, 22.6)
  line L34 (-23.0718, 22.6) -> (-26.5359, 28.6)
  line L35 (33.4641, 28.6) -> (26.5359, 28.6)
  line L36 (26.5359, 28.6) -> (23.0718, 22.6)
  line L37 (23.0718, 22.6) -> (26.5359, 16.6)
  line L38 (26.5359, 16.6) -> (33.4641, 16.6)
  line L39 (33.4641, 16.6) -> (36.9282, 22.6)
  line L40 (36.9282, 22.6) -> (33.4641, 28.6)
  line L41 (-26.5359, 45.2) -> (-33.4641, 45.2)
  line L42 (-33.4641, 45.2) -> (-36.9282, 39.2)
  line L43 (-36.9282, 39.2) -> (-33.4641, 33.2)
  line L44 (-33.4641, 33.2) -> (-26.5359, 33.2)
  line L45 (-26.5359, 33.2) -> (-23.0718, 39.2)
  line L46 (-23.0718, 39.2) -> (-26.5359, 45.2)
  line L47 (3.4641, 45.2) -> (-3.4641, 45.2)
  line L48 (-3.4641, 45.2) -> (-6.9282, 39.2)
  line L49 (-6.9282, 39.2) -> (-3.4641, 33.2)
  line L50 (-3.4641, 33.2) -> (3.4641, 33.2)
  line L51 (3.4641, 33.2) -> (6.9282, 39.2)
  line L52 (6.9282, 39.2) -> (3.4641, 45.2)
  line L53 (33.4641, 45.2) -> (26.5359, 45.2)
  line L54 (26.5359, 45.2) -> (23.0718, 39.2)
  line L55 (23.0718, 39.2) -> (26.5359, 33.2)
  line L56 (26.5359, 33.2) -> (33.4641, 33.2)
  line L57 (33.4641, 33.2) -> (36.9282, 39.2)
  line L58 (36.9282, 39.2) -> (33.4641, 45.2)
  point P0 (0, 22.6)
  dimension "d221" = 6
  dimension "d224" = 30
  dimension "d225" = 16.6
  constraint coincident L4.start origin
  constraint midpoint L2 L4.end
  constraint horizontal L9
  constraint coincident L4 P0
  constraint coincident L4.start L20
  measures "d221" distance of P0 L10
extrude "Extrude21" cut sketch "Sketch14" against normal blind 2.4 contours L5 L6 L7 L8 L9 L10 | L11 L12 L13 L14 L15 L16 | L17 L18 L19 L20 L21 L22 | L23 L24 L25 L26 L27 L28 | L29 L30 L31 L32 L33 L34 | L35 L36 L37 L38 L39 L40 | L41 L42 L43 L44 L45 L46 | L47 L48 L49 L50 L51 L52 | L53 L54 L55 L56 L57 L58 bodies 3 in component "M5xxx-base"
sketch "Sketch15" plane through (0, -78.4, 0) normal (0, -1, 0) x (1, 0, 0) in component "M5xxx-base"
  line L0 (65, 53.2) -> (88.8, 53.2)
  arc A0 (93.8, 48.2) -> (88.8, 53.2) centre (88.8, 48.2) ccw
  line L1 (93.8, 48.2) -> (93.8, 39.2)
  arc A1 (88.8, 34.2) -> (93.8, 39.2) centre (88.8, 39.2) ccw
  line L2 (88.8, 34.2) -> (65, 34.2)
  line L3 (65, 34.2) -> (65, 53.2)
  line L4 (64.6, 34.2) -> (41.2, 34.2)
  arc A2 (36.2, 39.2) -> (41.2, 34.2) centre (41.2, 39.2) ccw
  line L5 (36.2, 39.2) -> (36.2, 48.2)
  arc A3 (41.2, 53.2) -> (36.2, 48.2) centre (41.2, 48.2) ccw
  line L6 (41.2, 53.2) -> (64.6, 53.2)
  line L7 (64.6, 53.2) -> (64.6, 34.2)
  arc A4 (32.6, 42) -> (32.6, 45.8) centre (32.6, 43.9) ccw
  line L8 (32.6, 42) -> (21.4, 42)
  arc A5 (21.4, 45.8) -> (21.4, 42) centre (21.4, 43.9) ccw
  line L9 (21.4, 45.8) -> (32.6, 45.8)
  line L10 (-107, -6.1359) -> (106, -6.1359)
  line L11 (106, -6.1359) -> (106, 58.4)
  line L12 (106, 58.4) -> (-107, 58.4)
  line L13 (-107, 58.4) -> (-107, -6.1359)
  line L14 (-86.6077, 6) -> (-90.0718, 12)
  line L15 (-90.0718, 12) -> (-97, 12)
  line L16 (-97, 12) -> (-100.4641, 6)
  line L17 (-100.4641, 6) -> (-97, 0)
  line L18 (-97, 0) -> (-90.0718, 0)
  line L19 (-90.0718, 0) -> (-86.6077, 6)
  line L20 (-70.4641, 6) -> (-67, 0)
  line L21 (-67, 12) -> (-70.4641, 6)
  line L22 (-60.0718, 12) -> (-67, 12)
  line L23 (-56.6077, 6) -> (-60.0718, 12)
  line L24 (-60.0718, 0) -> (-56.6077, 6)
  line L25 (-67, 0) -> (-60.0718, 0)
  line L26 (-40.4641, 6) -> (-37, 0)
  line L27 (-37, 12) -> (-40.4641, 6)
  line L28 (-30.0718, 12) -> (-37, 12)
  line L29 (-26.6077, 6) -> (-30.0718, 12)
  line L30 (-30.0718, 0) -> (-26.6077, 6)
  line L31 (-37, 0) -> (-30.0718, 0)
  line L32 (-10.4641, 6) -> (-7, 0)
  line L33 (-7, 12) -> (-10.4641, 6)
  line L34 (-0.0718, 12) -> (-7, 12)
  line L35 (3.3923, 6) -> (-0.0718, 12)
  line L36 (-0.0718, 0) -> (3.3923, 6)
  line L37 (-7, 0) -> (-0.0718, 0)
  line L38 (-100.4641, 22.6) -> (-97, 16.6)
  line L39 (-97, 28.6) -> (-100.4641, 22.6)
  line L40 (-90.0718, 28.6) -> (-97, 28.6)
  line L41 (-86.6077, 22.6) -> (-90.0718, 28.6)
  line L42 (-90.0718, 16.6) -> (-86.6077, 22.6)
  line L43 (-97, 16.6) -> (-90.0718, 16.6)
  line L44 (-70.4641, 22.6) -> (-67, 16.6)
  line L45 (-67, 28.6) -> (-70.4641, 22.6)
  line L46 (-60.0718, 28.6) -> (-67, 28.6)
  line L47 (-56.6077, 22.6) -> (-60.0718, 28.6)
  line L48 (-60.0718, 16.6) -> (-56.6077, 22.6)
  line L49 (-67, 16.6) -> (-60.0718, 16.6)
  line L50 (-40.4641, 22.6) -> (-37, 16.6)
  line L51 (-37, 28.6) -> (-40.4641, 22.6)
  line L52 (-30.0718, 28.6) -> (-37, 28.6)
  line L53 (-26.6077, 22.6) -> (-30.0718, 28.6)
  line L54 (-30.0718, 16.6) -> (-26.6077, 22.6)
  line L55 (-37, 16.6) -> (-30.0718, 16.6)
  line L56 (-10.4641, 22.6) -> (-7, 16.6)
  line L57 (-7, 28.6) -> (-10.4641, 22.6)
  line L58 (-0.0718, 28.6) -> (-7, 28.6)
  line L59 (3.3923, 22.6) -> (-0.0718, 28.6)
  line L60 (-0.0718, 16.6) -> (3.3923, 22.6)
  line L61 (-7, 16.6) -> (-0.0718, 16.6)
  line L62 (-100.4641, 39.2) -> (-97, 33.2)
  line L63 (-97, 45.2) -> (-100.4641, 39.2)
  line L64 (-90.0718, 45.2) -> (-97, 45.2)
  line L65 (-86.6077, 39.2) -> (-90.0718, 45.2)
  line L66 (-90.0718, 33.2) -> (-86.6077, 39.2)
  line L67 (-97, 33.2) -> (-90.0718, 33.2)
  line L68 (-70.4641, 39.2) -> (-67, 33.2)
  line L69 (-67, 45.2) -> (-70.4641, 39.2)
  line L70 (-60.0718, 45.2) -> (-67, 45.2)
  line L71 (-56.6077, 39.2) -> (-60.0718, 45.2)
  line L72 (-60.0718, 33.2) -> (-56.6077, 39.2)
  line L73 (-67, 33.2) -> (-60.0718, 33.2)
  line L74 (-40.4641, 39.2) -> (-37, 33.2)
  line L75 (-37, 45.2) -> (-40.4641, 39.2)
  line L76 (-30.0718, 45.2) -> (-37, 45.2)
  line L77 (-26.6077, 39.2) -> (-30.0718, 45.2)
  line L78 (-30.0718, 33.2) -> (-26.6077, 39.2)
  line L79 (-37, 33.2) -> (-30.0718, 33.2)
  line L80 (-10.4641, 39.2) -> (-7, 33.2)
  line L81 (-7, 45.2) -> (-10.4641, 39.2)
  line L82 (-0.0718, 45.2) -> (-7, 45.2)
  line L83 (3.3923, 39.2) -> (-0.0718, 45.2)
  line L84 (-0.0718, 33.2) -> (3.3923, 39.2)
  line L85 (-7, 33.2) -> (-0.0718, 33.2)
  point P0 (-93.5359, 6)
  dimension "d228" = 6
  dimension "d229" = 10
  dimension "d232" = 30
  dimension "d233" = 16.6
  constraint horizontal L18
  constraint horizontal origin L18.end
  measures "d228" distance of P0 L19
  measures "d229" distance of L13 L17.end
extrude "Extrude22" cut sketch "Sketch15" against normal blind 156.8 contours L14 L15 L16 L17 L18 L19 | L20 L21 L22 L23 L24 L25 | L26 L27 L28 L29 L30 L31 | L32 L33 L34 L35 L36 L37 | L38 L39 L40 L41 L42 L43 | L44 L45 L46 L47 L48 L49 | L50 L51 L52 L53 L54 L55 | L56 L57 L58 L59 L60 L61 | L62 L63 L64 L65 L66 L67 | L68 L69 L70 L71 L72 L73 | L74 L75 L76 L77 L78 L79 | L80 L81 L82 L83 L84 L85 bodies 3 in component "M5xxx-base"
chamfer "Chamfer17" distance 2 angle 45 5 edges at (0, 72, -3.6) (107, 0, -3.6) (-45, -72, -3.6) (60, -72, -3.6) (-107, 0, -3.6) on bodies 3 in component "M5xxx-base"
ref_plane "WorkPlane1" through (-0.5072, 0, 58.4) normal (0, 0, 1) x (-1, 0, 0) in component "M5xxx-lid"
sketch "Sketch1 (3)" plane through (-0.5072, 0, 58.4) normal (0, 0, 1) x (1, 0, 0) in component "M5xxx-lid"
  arc A0 (-112.4928, -70) -> (-106.4928, -76) centre (-106.4928, -70) ccw
  line L0 (-112.4928, -70) -> (-112.4928, 70)
  arc A1 (-106.4928, 76) -> (-112.4928, 70) centre (-106.4928, 70) ccw
  line L1 (-106.4928, 76) -> (105.5072, 76)
  arc A2 (111.5072, 70) -> (105.5072, 76) centre (105.5072, 70) ccw
  line L2 (111.5072, 70) -> (111.5072, -70)
  arc A3 (105.5072, -76) -> (111.5072, -70) centre (105.5072, -70) ccw
  line L3 (105.5072, -76) -> (-106.4928, -76)
  line L4 (114.9072, -70) -> (114.9072, 70)
  arc A4 (114.9072, 70) -> (106.5072, 78.4) centre (106.5072, 70) ccw
  line L5 (106.5072, 78.4) -> (-106.4928, 78.4)
  arc A5 (-106.4928, 78.4) -> (-114.8928, 69.9653) centre (-106.4928, 70) ccw
  line L6 (-114.8928, 69.9653) -> (-114.8928, -69.9653)
  arc A6 (-114.8928, -69.9653) -> (-106.4928, -78.4) centre (-106.4928, -70) ccw
  line L7 (-106.4928, -78.4) -> (106.5072, -78.4)
  arc A7 (106.5072, -78.4) -> (114.9072, -70) centre (106.5072, -70) ccw
  line L8 (105.5072, -70) -> (-106.4928, -70)
  line L9 (105.5072, 70) -> (105.5072, -70)
  line L10 (-106.4928, 70) -> (105.5072, 70)
  line L11 (-106.4928, -70) -> (-106.4928, 70)
  dimension "d278" = 6
extrude "Extrude2''" add sketch "Sketch1 (3)" against normal blind 4 separate body contours A0 L0 A1 L1 A2 L2 A3 L3 makes body 4 in component "M5xxx-lid"
extrude "Extrude1'''" add sketch "Sketch1 (3)" along normal blind 2.4 contours A0 L0 A1 L1 A2 L2 A3 L3 | L4 A4 L5 A5 L6 A6 L7 A7 | L8 L9 L10 L11 bodies 4 in component "M5xxx-lid"
fillet "Fillet1''" radius 2.5 4 edges at (105, 70, 56.4) (-107, 70, 56.4) (105, -70, 56.4) (-107, -70, 56.4) on bodies 4 in component "M5xxx-lid"